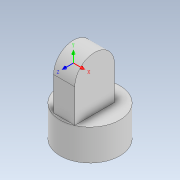
# Autodesk Inventor part: hip_back
Saved by Autodesk Inventor 2020 (Build 240168000, 168)
## iProperties
Created: 2021-01-29
Part Number: hip_back
Material: Generic
Document SubType Name: Modeling
Designer: DELL
Density: 1 g/cm^3
Appearance: Default
Author: DELL
Autodesk Inventor part; units mm, degrees
ref_plane "YZ Plane" through (0, 0, 0) normal (1, 0, 0) x (0, 1, 0)
ref_plane "XZ Plane" through (0, 0, 0) normal (0, 1, 0) x (-1, 0, 0)
sketch "Sketch1" plane through (0, 0, 0) normal (1, 0, 0) x (0, 1, 0)
  circle A0 centre (0, 0) radius 30
  line L0 (0, 30) -> (-50.5, 30)
  line L1 (-50.5, 30) -> (-50.5, -30)
  line L2 (-50.5, -30) -> (0, -30)
  dimension "d0" = 60
  dimension "d1" = 50.5
  constraints: 6 end point, 2 perpendicular, 2 point on circle, 2 tangent, 1 centre point, 1 coincident, 1 horizontal
  measures "d0" diameter of A0
  measures "d1" distance of L0.start L0.end
extrude "Extrusion1" add sketch "Sketch1" along normal blind 32
sketch "Sketch2" plane through (0, -50.5, -30) normal (0, -1, 0) x (1, 0, 0)
  circle A0 centre (14, 19) radius 45
  line L0 (0, 60) -> (32, 60) projected
  line L1 (0, 60) -> (0, 0) projected
  line L2 (0, 0) -> (0, 60) projected
  line L3 (0, 60) -> (32, 60) projected
  line L4 (32, 0) -> (32, 60) projected
  line L5 (0, 0) -> (32, 0) projected
  line L6 (0, 30) -> (32, 30) construction
  point P0 (16, 60)
  point P1 (0, 30)
  dimension "d5" = 90
  dimension "d18" = 11
  dimension "d19" = 14
  constraints: 3 midpoint, 2 end point, 1 centre point, 1 horizontal
  measures "d5" diameter of A0
  measures "d18" distance from line of A0.centre L6
  measures "d19" distance from line of L1 A0.centre
extrude "Extrusion2" add sketch "Sketch2" along normal blind 47 contours A0 | L0 L4 L5 L1
ref_plane "Work Plane1" through (0, -74, -30) normal (0, 1, 0) x (1, 0, 0)
sketch "Sketch3" plane through (14, -97.5, -11) normal (0, -1, 0) x (1, 0, 0)
  circle A0 centre (0, 0) radius 45 projected
  circle A1 centre (0, 0) radius 40
  line L0 (0, 0) -> (-45, 0) construction
  line L1 (0, 0) -> (-38.9711, 22.5) construction
  line L2 (0, 0) -> (-38.9711, -22.5) construction
  line L3 (-34.641, 20) -> (-24.3333, 37.8536)
  line L4 (-34.641, -20) -> (-24.3333, -37.8536)
  point P0 (-14, 11)
  dimension "d14" = 80
  dimension "d15" = 30
  constraints: 10 end point, 7 point on circle, 2 point on line, 2 tangent, 1 centre point, 1 coincident, 1 horizontal, 1 other
  measures "d14" diameter of A1
  measures "d15" angle of L0 L1
body "Solid1"
